Autodesk Inventor part; units mm, degrees
(part 2 of 2)
sketch "Sketch16" plane through (-93.3464, 30, 62.7) normal (0, 0, 1) x (1, 0, 0)
  line L0 (6.6464, 0) -> (6.6464, -15) projected
  line L1 (160.0464, -15) -> (160.0464, 0) projected
  line L2 (166.6929, 0) -> (166.6929, -23) projected
  line L3 (0, 0) -> (166.6929, 0) projected
  line L4 (0, -23) -> (0, 0) projected
  line L5 (166.6929, -23) -> (0, -23) projected
  line L6 (160.0464, 0) -> (6.6464, 0) projected
  line L7 (6.6464, -15) -> (160.0464, -15) projected
  line L8 (6.6464, -7.5) -> (45.8464, -7.5) construction
  arc A0 (40.3464, -7.5) -> (45.8464, -13) centre (45.8464, -7.5) ccw
  arc A1 (120.8464, -13) -> (126.3464, -7.5) centre (120.8464, -7.5) ccw
  line L9 (40.3464, -7.5) -> (40.3464, 0)
  line L10 (40.3464, 0) -> (51.3464, 0)
  line L11 (115.3464, 0) -> (126.3464, 0)
  line L12 (126.3464, -7.5) -> (126.3464, 0)
  line L13 (45.8464, -13) -> (120.8464, -13)
  line L14 (40.3464, 0) -> (126.3464, 0)
  line L15 (40.3464, 0) -> (126.3464, 0)
  point P0 (93.3464, -30)
  point P1 (65.3464, -7.5)
  point P2 (76.3464, -7.5)
  point P3 (90.8464, -7.5)
  point P4 (100.8464, -7.5)
  point P5 (126.3464, 0)
  point P6 (40.3464, 0)
  point P7 (40.3464, 0)
  point P8 (51.3464, 0)
  point P9 (115.3464, 0)
  point P10 (126.3464, 0)
  dimension "d241" = 153.4
  dimension "d242" = 39.2
  dimension "d243" = 11
  dimension "d249" = 11
  constraints: 16 end point, 5 point on line, 4 point on circle, 2 centre point, 2 collinear, 2 perpendicular, 2 tangent, 1 coincident, 1 horizontal, 1 midpoint
  measures "d241" distance between parallel lines of L1 L0
  measures "d242" distance of L8.start L8.end
  measures "d243" diameter of A0
  measures "d249" diameter of A1
extrude "Extrusion17" cut sketch "Sketch16" against normal through all contours L3 L12 A1 L13 A0 L9
body "Solid1"
